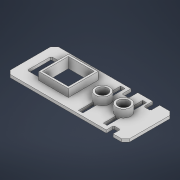
# Autodesk Inventor part: Interface shield
Saved by Autodesk Inventor 2021 (Build 250183000, 183)
## iProperties
Created: 2021-06-30
Part Number: Interface shield
Material: Generic
Document SubType Name: Modeling
Designer: allen
Density: 1 g/cm^3
Appearance: Default
Author: allen
Autodesk Inventor part; units mm, degrees
ref_plane "YZ Plane" through (0, 0, 0) normal (1, 0, 0) x (0, 1, 0)
ref_plane "XZ Plane" through (0, 0, 0) normal (0, 1, 0) x (-1, 0, 0)
ref_plane "XY Plane" through (0, 0, 0) normal (0, 0, 1) x (1, 0, 0)
sketch "Sketch1" plane through (0, 0, 0) normal (0, 1, 0) x (-1, 0, 0)
  line L0 (0, 0) -> (-62, 0)
  line L1 (-62, 0) -> (-62, -25)
  line L2 (-62, -25) -> (0, -25)
  line L3 (0, -25) -> (0, 0)
  dimension "d0" = 62
  dimension "d1" = 25
  constraints: 8 end point, 2 parallel, 1 horizontal, 1 perpendicular
  measures "d0" distance of L1.end L2.end
  measures "d1" distance of L2.end L0.start
extrude "Extrusion1" add sketch "Sketch1" along normal blind 1.5
sketch "Sketch2" plane through (0, 1.5, 0) normal (0, 1, 0) x (1, 0, 0)
  line L0 (62, 0) -> (62, 25) projected
  point P0 (0, 0)
  point P1 (37.5, 12.5)
  point P2 (48.5, 12.5)
  point P3 (62, 12.5)
  dimension "d4" = 11
  dimension "d5" = 13.5
  constraints: 2 horizontal alignment, 1 midpoint
  measures "d4" distance of point (48.5, 12.5) point (37.5, 12.5)
  measures "d5" distance from line of L0 point (48.5, 12.5)
hole "Hole1" at (37.5, 1.5, -12.5) at (48.5, 1.5, -12.5) direction (0, -1, 0) diameter 5.5 end through all
sketch "Sketch3" plane through (0, 1.5, 0) normal (0, 1, 0) x (1, 0, 0)
  circle A0 centre (37.5, 12.5) radius 2.75 projected
  circle A1 centre (48.5, 12.5) radius 2.75 projected
  circle A2 centre (37.5, 12.5) radius 3.75
  circle A3 centre (48.5, 12.5) radius 3.75
  point P0 (0, 0)
  dimension "d13" = 1
  dimension "d14" = 1
  constraints: 2 centre point
  measures "d13" radial gap between concentric circles of A0 A2
  measures "d14" radial gap between concentric circles of A1 A3
extrude "Extrusion2" add sketch "Sketch3" along normal blind 4
sketch "Sketch4" plane through (0, 0, 0) normal (0, -1, 0) x (1, 0, 0)
  circle A0 centre (37.5, -12.5) radius 2.75 construction
  circle A1 centre (48.5, -12.5) radius 2.75 construction
  circle A2 centre (37.5, -12.5) radius 3.1
  circle A3 centre (48.5, -12.5) radius 3.1
  point P0 (0, 0)
  dimension "d17" = 6.2
  constraints: 2 centre point, 1 equal radius
  measures "d17" diameter of A2
emboss "Emboss1" sketch "Sketch4" operation cut depth 0.5 direction (0, 1, 0)
sketch "Sketch5" plane through (0, 1.5, 0) normal (0, 1, 0) x (1, 0, 0)
  line L0 (13, 19.25) -> (26.5, 19.25)
  line L1 (26.5, 19.25) -> (26.5, 5.75)
  line L2 (26.5, 5.75) -> (13, 5.75)
  line L3 (13, 5.75) -> (13, 19.25)
  circle A0 centre (37.5, 12.5) radius 2.75 construction
  point P0 (0, 0)
  point P1 (26.5, 12.5)
  dimension "d20" = 11
  dimension "d21" = 13.5
  constraints: 8 end point, 2 parallel, 2 perpendicular, 1 horizontal, 1 horizontal alignment, 1 midpoint
  measures "d20" distance from line of A0.centre L1
  measures "d21" distance of L0.end L1.end
extrude "Extrusion3" cut sketch "Sketch5" against normal through all
sketch "Sketch6" plane through (0, 1.5, 0) normal (0, 1, 0) x (1, 0, 0)
  line L0 (13, 19.25) -> (26.5, 19.25) projected
  line L1 (26.5, 19.25) -> (26.5, 5.75) projected
  line L2 (13, 5.75) -> (13, 19.25) projected
  line L3 (26.5, 5.75) -> (13, 5.75) projected
  line L4 (27.5, 20.25) -> (12, 20.25)
  line L5 (12, 20.25) -> (12, 4.75)
  line L6 (12, 4.75) -> (27.5, 4.75)
  line L7 (27.5, 4.75) -> (27.5, 20.25)
  point P0 (0, 0)
  dimension "d24" = 1
  constraints: 8 end point, 3 other
  measures "d24" distance between parallel lines of L1 L7
extrude "Extrusion4" add sketch "Sketch6" along normal up to surface (4 mm away)
sketch "Sketch7" plane through (0, 1.5, 0) normal (0, 1, 0) x (1, 0, 0)
  circle A0 centre (37.5, 12.5) radius 3.75 projected
  circle A1 centre (48.5, 12.5) radius 3.75 projected
  line L0 (62, 25) -> (0, 25) projected
  line L1 (37.5, 25) -> (37.5, 0) construction
  line L2 (0, 0) -> (62, 0) projected
  line L3 (38.25, 23.5) -> (38.25, 1.5)
  line L4 (36, 23.5) -> (36, 1.5)
  line L5 (41.25, 12.5) -> (44.75, 12.5) construction
  line L6 (36, 23.5) -> (38.25, 23.5)
  line L7 (12, 20.25) -> (27.5, 20.25) projected
  line L8 (36, 1.5) -> (38.25, 1.5)
  line L9 (48.2, 22.75) -> (48.2, 2.25)
  line L10 (50.2, 22.75) -> (50.2, 2.25)
  line L11 (50.2, 22.75) -> (48.2, 22.75)
  line L12 (50.2, 2.25) -> (48.2, 2.25)
  point P0 (49.2, 12.5)
  point P1 (50.2, 9.1575)
  point P2 (48.2, 8.762)
  point P3 (48.2, 16.238)
  point P4 (50.2, 15.8425)
  point P5 (38.25, 8.8258)
  point P6 (36, 9.0631)
  point P7 (36, 15.9369)
  point P8 (38.25, 16.1742)
  point P9 (49.2, 22.75)
  point P10 (50.2, 12.5)
  dimension "d28" = 0.75
  dimension "d30" = 3.25
  dimension "d61" = 0.7
  dimension "d62" = 20.5
  dimension "d63" = 2
  dimension "d64" = 1.5
  constraints: 20 end point, 3 horizontal, 3 horizontal alignment, 3 vertical, 2 midpoint, 2 parallel, 2 point on line, 2 symmetric about line, 2 vertical alignment, 1 perpendicular, 4 other
  measures "d28" distance between parallel lines of L1 L3
  measures "d30" distance between parallel lines of L7 L6
  measures "d61" distance of point (49.2, 12.5) point (48.5, 12.5)
  measures "d62" distance of L11.start L12.start
  measures "d63" distance of L11.start L11.end
  measures "d64" distance between parallel lines of L1 L4
extrude "Extrusion5" cut sketch "Sketch7" against normal through all contours A0 L4 L6 L3 | L3 L8 L4 A0 | A1 L9 L11 L10 | L10 L12 L9 A1
sketch "Sketch8" plane through (0, 1.5, 0) normal (0, 1, 0) x (1, 0, 0)
  line L0 (62, 25) -> (0, 25) projected
  line L1 (39.875, 25) -> (43.375, 25)
  line L2 (43.375, 25) -> (43.375, 20.25)
  line L3 (43.375, 20.25) -> (39.875, 20.25)
  line L4 (39.875, 20.25) -> (39.875, 25)
  line L5 (36, 23.5) -> (38.25, 23.5) projected
  line L6 (51.25, 25) -> (54.75, 25)
  line L7 (54.75, 25) -> (54.75, 20.25)
  line L8 (54.75, 20.25) -> (51.25, 20.25)
  line L9 (51.25, 20.25) -> (51.25, 25)
  line L10 (50.2, 22.75) -> (48.2, 22.75) projected
  line L11 (52, 0) -> (55.5, 0)
  line L12 (55.5, 0) -> (55.5, 3.8)
  line L13 (55.5, 3.8) -> (52, 3.8)
  line L14 (52, 3.8) -> (52, 0)
  line L15 (50.2, 2.25) -> (48.2, 2.25) projected
  line L16 (0, 0) -> (62, 0) projected
  circle A0 centre (48.5, 12.5) radius 2.75 construction
  line L17 (12, 20.25) -> (27.5, 20.25) projected
  point P0 (41.625, 20.25)
  point P1 (37.125, 23.5)
  point P2 (49.2, 22.75)
  point P3 (53, 20.25)
  point P4 (54.75, 25)
  dimension "d33" = 4.5
  dimension "d34" = 3.5
  dimension "d53" = 0.75
  dimension "d54" = 3.5
  dimension "d57" = 3.8
  dimension "d60" = 4.5
  constraints: 24 end point, 6 parallel, 4 midpoint, 3 horizontal, 3 perpendicular, 2 collinear, 2 equal length, 2 point on line
  measures "d33" horizontal distance of point (41.625, 20.25) point (37.125, 23.5)
  measures "d34" distance of L2.end L3.end
  measures "d53" distance between parallel lines of L14 L9
  measures "d54" distance between parallel lines of L12 L14
  measures "d57" distance between parallel lines of L16 L13
  measures "d60" horizontal distance of point (53, 20.25) A0.centre
extrude "Extrusion6" cut sketch "Sketch8" against normal through all
sketch "Sketch9" plane through (0, 0, 0) normal (0, -1, 0) x (1, 0, 0)
  arc A0 (36, -15.9369) -> (38.25, -16.1742) centre (37.5, -12.5) ccw projected
  line L0 (36, -1.5) -> (36, -9.0631) construction
  line L1 (36, -15.9369) -> (36, -9.0631)
  arc A1 (38.25, -16.1742) -> (38.25, -8.8258) centre (37.5, -12.5) ccw construction
  line L2 (38.25, -16.1742) -> (38.25, -8.8258)
  arc A2 (38.25, -8.8258) -> (36, -9.0631) centre (37.5, -12.5) ccw projected
  arc A3 (48.2, -16.238) -> (50.2, -15.8425) centre (48.5, -12.5) ccw projected
  arc A4 (48.2, -8.762) -> (48.2, -16.238) centre (48.5, -12.5) ccw construction
  line L3 (48.2, -16.238) -> (48.2, -8.762)
  line L4 (50.2, -9.1575) -> (50.2, -2.25) construction
  line L5 (50.2, -9.1575) -> (50.2, -15.8425)
  arc A5 (50.2, -9.1575) -> (48.2, -8.762) centre (48.5, -12.5) ccw projected
  point P0 (0, 0)
  constraints: 8 end point, 3 vertical, 1 collinear
extrude "Extrusion7" cut sketch "Sketch9" against normal up to surface (0.5 mm away)
sketch "Sketch10" plane through (0, 1.5, 0) normal (0, 1, 0) x (1, 0, 0)
  line L0 (4.5, 18.75) -> (11.5, 18.75)
  line L1 (11.5, 18.75) -> (11.5, 6.25)
  line L2 (11.5, 6.25) -> (4.5, 6.25)
  line L3 (4.5, 6.25) -> (4.5, 18.75)
  line L4 (0, 25) -> (0, 0) projected
  line L5 (26.5, 19.25) -> (13, 19.25) projected
  line L6 (13, 5.75) -> (26.5, 5.75) projected
  point P0 (4.5, 12.5)
  point P1 (0, 12.5)
  dimension "d40" = 7
  dimension "d41" = 4.5
  dimension "d58" = 12.5
  constraints: 8 end point, 2 midpoint, 2 parallel, 1 horizontal, 1 horizontal alignment, 1 perpendicular
  measures "d40" distance of L1.end L2.end
  measures "d41" distance between parallel lines of L4 L3
  measures "d58" distance between parallel lines of L2 L0
extrude "Extrusion8" cut sketch "Sketch10" against normal through all
chamfer "Chamfer1" distance 0.5 angle 45 10 edges at (4.5, 0.75, -18.75) (11.5, 0.75, -18.75) (4.5, 0.75, -6.25) (11.5, 0.75, -6.25) (39.875, 0.75, -20.25) (43.375, 0.75, -20.25) (54.75, 0.75, -20.25) (51.25, 0.75, -20.25) (55.5, 0.75, -3.8) (52, 0.75, -3.8)
chamfer "Chamfer2" distance 0.1 angle 45 8 edges at (50.2, 0.75, -2.25) (48.2, 0.75, -2.25) (50.2, 0.75, -22.75) (48.2, 0.75, -22.75) (38.25, 0.75, -23.5) (36, 0.75, -23.5) (38.25, 0.75, -1.5) (36, 0.75, -1.5)
chamfer "Chamfer3" distance 2 angle 45 4 edges at (62, 0.75, -25) (62, 0.75, 0) (0, 0.75, -25) (0, 0.75, 0)
equation "\"d54\" = d34"
equation "\"d57\" = d55"
equation "\"d55\" = 3.8"
body "Solid1"
